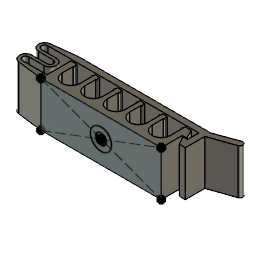
Cable Organizer V3 (Autodesk Fusion 360 design; units mm, degrees)
Autodesk Fusion 360 part; units mm, degrees
sketch "Sketch1" plane through (0, 0, 0) normal (0, 0, 1) x (1, 0, 0)
  line L0 (-5, 5) -> (35, 5)
  line L1 (35, 5) -> (35, -5)
  line L2 (35, -5) -> (-5, -5)
  line L3 (-5, -5) -> (-5, 5)
  arc A0 (-3, 0) -> (3, 0) centre (0, 0) ccw
  arc A1 (-3, 3.7) -> (-3, 4.3) centre (-3, 4) ccw
  arc A2 (3, 4.3) -> (3, 3.7) centre (3, 4) ccw
  line L4 (-3, 0) -> (-3, 3.7)
  line L5 (-3, 4.3) -> (-3, 5)
  line L6 (3, 0) -> (3, 3.7)
  line L7 (3, 4.3) -> (3, 5)
  line L8 (4.5, 4.3) -> (4.5, 5)
  arc A3 (4.5, 3.7) -> (4.5, 4.3) centre (4.5, 4) ccw
  line L9 (4.5, 0) -> (4.5, 3.7)
  arc A4 (4.5, 0) -> (10.5, 0) centre (7.5, 0) ccw
  line L10 (10.5, 0) -> (10.5, 3.7)
  arc A5 (10.5, 4.3) -> (10.5, 3.7) centre (10.5, 4) ccw
  line L11 (10.5, 4.3) -> (10.5, 5)
  line L12 (12, 4.3) -> (12, 5)
  arc A6 (12, 3.7) -> (12, 4.3) centre (12, 4) ccw
  line L13 (12, 0) -> (12, 3.7)
  arc A7 (12, 0) -> (18, 0) centre (15, 0) ccw
  line L14 (18, 0) -> (18, 3.7)
  arc A8 (18, 4.3) -> (18, 3.7) centre (18, 4) ccw
  line L15 (18, 4.3) -> (18, 5)
  line L16 (19.5, 4.3) -> (19.5, 5)
  arc A9 (19.5, 3.7) -> (19.5, 4.3) centre (19.5, 4) ccw
  line L17 (19.5, 0) -> (19.5, 3.7)
  arc A10 (19.5, 0) -> (25.5, 0) centre (22.5, 0) ccw
  line L18 (25.5, 0) -> (25.5, 3.7)
  arc A11 (25.5, 4.3) -> (25.5, 3.7) centre (25.5, 4) ccw
  line L19 (25.5, 4.3) -> (25.5, 5)
  line L20 (27, 4.3) -> (27, 5)
  arc A12 (27, 3.7) -> (27, 4.3) centre (27, 4) ccw
  line L21 (27, 0) -> (27, 3.7)
  arc A13 (27, 0) -> (33, 0) centre (30, 0) ccw
  line L22 (33, 0) -> (33, 3.7)
  arc A14 (33, 4.3) -> (33, 3.7) centre (33, 4) ccw
  line L23 (33, 4.3) -> (33, 5)
  line L24 (39, 5.5) -> (-5, 5.5)
  line L25 (-5, 5.5) -> (-5, 7.5) construction
  line L26 (-5, 7.5) -> (39, 7.5)
  line L27 (39, 7.5) -> (39, 5.5) construction
  line L28 (-13.1667, -0.8333) -> (-8.1667, -0.8333)
  line L29 (-13.1667, 0.1667) -> (-8.1667, 0.1667)
  line L30 (-13.1667, 2.3333) -> (-8.1667, 2.3333)
  line L31 (-13.1667, 3.3333) -> (-8.1667, 3.3333)
  line L32 (-13.4161, -3.985) -> (-5, -5)
  line L33 (-13.1667, 5.5) -> (-5, 5.5)
  line L34 (-13.1667, -3) -> (-5, -3)
  line L35 (-13.4161, 6.485) -> (-5, 7.5)
  arc A15 (-13.1667, 5.5) -> (-13.1667, 3.3333) centre (-13.1667, 4.4167) ccw
  arc A16 (-8.1667, 0.1667) -> (-8.1667, 2.3333) centre (-8.1667, 1.25) ccw
  arc A17 (-13.1667, -0.8333) -> (-13.1667, -3) centre (-13.1667, -1.9167) ccw
  arc A18 (-13.1667, 0.1667) -> (-13.4161, -3.985) centre (-13.1667, -1.9167) ccw
  arc A19 (-8.1667, -0.8333) -> (-8.1667, 3.3333) centre (-8.1667, 1.25) ccw
  arc A20 (-13.4161, 6.485) -> (-13.1667, 2.3333) centre (-13.1667, 4.4167) ccw
  line L36 (39, 7.5) -> (46.5175, 10.2362)
  line L37 (46.5175, 10.2362) -> (47.2016, 8.3568) construction
  arc A21 (47.2016, 8.3568) -> (46.5175, 10.2362) centre (46.8596, 9.2965) ccw
  line L38 (39, 5.5) -> (47.2016, 8.3568)
  line L39 (39, 5.5) -> (37, 5.5) construction
  line L40 (37, 5.5) -> (37, -1)
  line L41 (37, -1) -> (39, -1)
  line L42 (39, -1) -> (39, 5.5)
  line L43 (35, 2) -> (36.0955, 2)
  line L44 (37, 1.75) -> (35.9211, 1.75)
  line L45 (35.7017, 1.3803) -> (37, -1)
  line L46 (36.3191, 2.3618) -> (35, 5)
  arc A22 (35.9211, 1.75) -> (35.7017, 1.3803) centre (35.9211, 1.5) ccw
  arc A23 (36.0955, 2) -> (36.3191, 2.3618) centre (36.0955, 2.25) ccw
  point P0 (36.5, 2)
  point P1 (35.5, 1.75)
  dimension "d5" = 6
  dimension "d11" = 5
  dimension "d12" = 5
  dimension "d13" = 5
  dimension "d14" = 35
  dimension "d15" = 0.6
  dimension "d16" = 1
  dimension "d17" = 0.6
  dimension "d18" = 1
  dimension "d21" = 7.5
  dimension "d22" = 0
  dimension "d23" = 2
  dimension "d24" = 0.5
  dimension "d25" = 40
  dimension "d26" = 44
  dimension "d28" = 2.1667
  dimension "d29" = 2.1667
  dimension "d30" = 2.1667
  dimension "d31" = 3.0833
  dimension "d33" = 3.1667
  dimension "d34" = 3.1667
  dimension "d35" = 8.1667
  dimension "d36" = 8.1667
  dimension "d37" = 3.1667
  dimension "d38" = 4.1667
  dimension "d39" = 4.1667
  dimension "d40" = 4.1667
  dimension "d41" = 8
  dimension "d43" = 160
  dimension "d45" = 2
  dimension "d46" = 90
  dimension "d48" = 2
  dimension "d49" = 6.5
  dimension "d50" = 1.5
  dimension "d51" = 3
  dimension "d52" = 1.5
  dimension "d53" = 2.75
  dimension "d55" = 0.25
  dimension "d56" = 0.25
  constraint coincident A0.centre origin
  constraint horizontal L0
  constraint vertical L1
  constraint horizontal L2
  constraint vertical L3
  constraint tangent A0 L4
  constraint coincident L0 L5.end
  constraint perpendicular L0 L4
  constraint tangent A0 L6
  constraint coincident L0 L7.end
  constraint perpendicular L0 L6
  constraint coincident A1.centre L4
  constraint coincident A2.centre L6
  constraint coincident A1.end L4
  constraint coincident A2.start L6
  constraint collinear L4 L5
  constraint collinear L6 L7
  constraint horizontal L24
  constraint vertical L25
  constraint horizontal L26
  constraint vertical L27
  constraint concentric A15 A20
  constraint concentric A16 A19
  constraint concentric A17 A18
  constraint tangent L28 A17
  constraint tangent L28 A19
  constraint tangent L29 A18
  constraint tangent L29 A16
  constraint tangent L30 A20
  constraint tangent L30 A16
  constraint tangent L31 A15
  constraint tangent L31 A19
  constraint tangent L32 A18
  constraint tangent L33 A15
  constraint tangent L34 A17
  constraint coincident L3 L34.end
  constraint perpendicular L3 L34
  constraint tangent L35 A20
  constraint tangent L36 A21
  constraint vertical L0.start L24.end
  constraint horizontal L39
  constraint vertical L40
  constraint horizontal L41
  constraint vertical L42
  constraint coincident L1 L43.start
  constraint perpendicular L1 L43
  constraint coincident L40 L44.start
  constraint perpendicular L40 L44
  constraint coincident P1 L44
  constraint coincident P1 L45
  constraint tangent L44 A22
  constraint tangent L45 A22
  constraint coincident P0 L43
  constraint coincident P0 L46
  constraint tangent L43 A23
  constraint tangent L46 A23
  measures "d5" diameter of A0
  measures "d11" distance of A0.centre L2
  measures "d12" distance of A0.centre L0
  measures "d13" distance of A0.centre L3
  measures "d14" distance of A0.centre L1
  measures "d15" diameter of A1
  measures "d16" distance of L0 A1.centre
  measures "d17" diameter of A2
  measures "d18" distance of L0 A2.centre
  measures "d23" distance of L24 L26
  measures "d24" distance of L0 L24
  measures "d25" distance of L1 L3
  measures "d26" distance of L25 L27
  measures "d28" diameter of A16
  measures "d29" diameter of A15
  measures "d30" diameter of A17
  measures "d31" distance of L2 A17.centre
  measures "d33" vertical distance of A16.centre A17.centre
  measures "d34" vertical distance of A15.centre A16.centre
  measures "d35" distance of L3 A17.centre
  measures "d36" distance of L3 A15.centre
  measures "d37" distance of L3 A16.centre
  measures "d38" diameter of A20
  measures "d39" diameter of A19
  measures "d40" diameter of A18
  measures "d41" distance of L26.end L36.end
  measures "d43" angle of L26 L36
  measures "d45" distance of L36.end L37.end
  measures "d46" angle of L36 L37
  measures "d48" distance of L24.start L39.end
  measures "d49" distance of L24.start L41.end
  measures "d50" distance of L43.start P0
  measures "d51" distance of L0.end L43
  measures "d52" distance of L44.start P1
  measures "d53" distance of L41 L44
  measures "d55" radius of A22
  measures "d56" radius of A23
extrude "Extrude1" add sketch "Sketch1" along normal blind 15 contours L0 L1 L2 L3 A0 A1 A2 L4 L5 L6 L7 L8 A3 L9 A4 L10 A5 L11 L12 A6 L13 A7 L14 A8 L15 L16 A9 L17 A10 L18 A11 L19 L20 A12 L21 A13 L22 A14 L23 | L3 L24 L26 L28 L29 L30 L31 L32 L33 L34 L35 A15 A16 A17 A18 A19 A20 L36 A21 L38 | L1 L43 L46 A23 | L24 L40 L41 L42 | L40 L44 L45 A22
sketch "Sketch2" plane through (0, -5, 0) normal (0, -1, 0) x (1, 0, 0)
  line L0 (-5, 0) -> (35, 0)
  line L1 (35, 0) -> (35, 15)
  line L2 (35, 15) -> (-5, 15)
  line L3 (-5, 15) -> (-5, 0)
  circle A0 centre (15, 7.5) radius 1.75
  line L4 (-5, 15) -> (35, 0) construction
  line L5 (-5, 0) -> (35, 15) construction
  circle A1 centre (15, 7.5) radius 3.5
  dimension "d60" = 3.5
  dimension "d63" = 7
  constraint coincident L2.end L3.start
  constraint coincident L0.end L1.start
  constraint coincident L0.start L3.end
  constraint coincident L1.end L2.start
  constraint coincident A0.centre L4
  constraint coincident A0.centre L5
  constraint concentric A0 A1
  measures "d60" diameter of A0
  measures "d63" diameter of A1
extrude "Extrude2" cut sketch "Sketch2" against normal blind 5 contours A0
extrude "Extrude3" cut sketch "Sketch2" along normal blind -2 and the other way blind 10 contours A1
chamfer "Chamfer1" distance 1.75 angle 45 1 edges at (13.3684, -3, 8.1328)
equation "Diameter = 6 mm"
equation "HolesSpacing = 1.5 mm"
equation "NotchSize = 0.3 mm"
equation "HolesNumber = 5"
equation "d5 = Diameter"
equation "Thickness = 2 mm"
equation "d11 = Diameter / 2 + Thickness"
equation "d12 = Diameter / 2 + Thickness"
equation "d13 = Diameter / 2 + Thickness"
equation "d14 = ( Diameter + HolesSpacing ) * HolesNumber - ( Diameter / 2 ) + Thickness - HolesSpacing"
equation "d15 = NotchSize * 2"
equation "d16 = Thickness / 2"
equation "d17 = NotchSize * 2"
equation "d18 = Thickness / 2"
equation "d19 = HolesNumber"
equation "d21 = Diameter + HolesSpacing"
equation "d23 = Thickness"
equation "d24 = Spacing"
equation "d26 = d25 + Thickness * 2"
equation "d28 = d30"
equation "d29 = d30"
equation "d30 = ( Thickness + Diameter + Spacing - Thickness ) / 3"
equation "d31 = d30 / 2 + Thickness"
equation "d33 = d30 + Thickness / 2"
equation "d34 = d30 + Thickness / 2"
equation "d35 = d30 + Diameter"
equation "d36 = d30 + Diameter"
equation "d37 = d30 + Thickness / 2"
equation "d38 = d30 + Thickness"
equation "d39 = d30 + Thickness"
equation "d40 = d30 + Thickness"
equation "d41 = Diameter + Thickness"
equation "d45 = Thickness"
equation "Spacing = 0.5 mm"
equation "d48 = Thickness"
equation "d49 = Diameter + Spacing"
equation "d50 = Thickness * 3 / 4"
equation "d51 = Diameter / 2"
equation "d52 = Thickness * 3 / 4"
equation "d53 = Diameter / 2 - Spacing / 2"
equation "Fillet = 0.25 mm"
equation "d55 = Fillet"
equation "d56 = Fillet"
equation "d57 = Width"
equation "Width = 15 mm"
equation "d60 = ScrewThread"
equation "ScrewThread = 3.5 mm"
equation "ScrewHead = 7 mm"
equation "d63 = ScrewHead"
equation "d64 = -Thickness - Diameter / 2"
equation "d66 = -Thickness"
equation "d68 = 2 * Thickness + Diameter"
equation "d70 = Thickness * 3.5 / 4"
